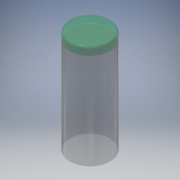
# Autodesk Inventor part: Jar
Saved by Autodesk Inventor 2019 (Build 230136000, 136)
## iProperties
Created: 2018-12-14
Part Number: Jar
Material: Polycarbonate, Clear
Document SubType Name: Modeling
Designer: assman
Density: 1.2 g/cm^3
Appearance: Polycarbonate - Clear
Author: assman
Autodesk Inventor part; units mm, degrees
ref_plane "YZ Plane" through (0, 0, 0) normal (1, 0, 0) x (0, 1, 0)
ref_plane "XZ Plane" through (0, 0, 0) normal (0, 1, 0) x (-1, 0, 0)
ref_plane "XY Plane" through (0, 0, 0) normal (0, 0, 1) x (1, 0, 0)
sketch "Sketch1" plane through (0, 0, 0) normal (0, 1, 0) x (-1, 0, 0)
  circle A0 centre (0, 0) radius 52
  dimension "d0" = 104
  constraints: 1 centre point, 1 coincident
  measures "d0" diameter of A0
extrude "Extrusion1" add sketch "Sketch1" along normal blind 245
shell "Shell1" thickness 1.5 removed faces 1 at (-18.5271, 0, 25.061)
sketch "Sketch2" plane through (0, 245, 0) normal (0, 1, 0) x (1, 0, 0)
  circle A0 centre (0, 0) radius 52 projected
  circle A1 centre (0, 0) radius 52
  constraints: 1 centre point, 1 coincident
extrude "Extrusion2" add sketch "Sketch2" along normal blind 20 separate body
fillet "Fillet1" radius 5 1 edges at (-52, 265, 0)
body "Solid1"
body "Solid2"
